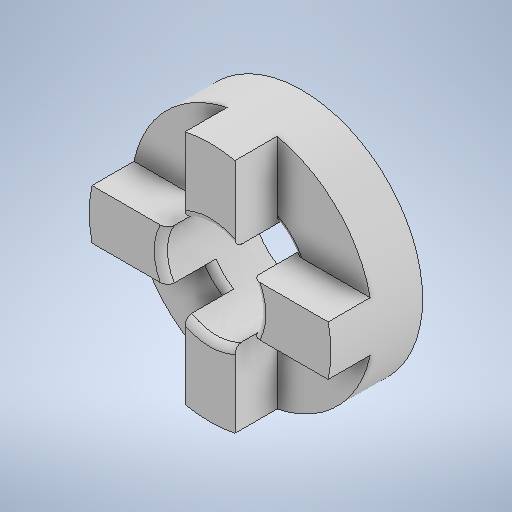
# Autodesk Inventor part: trava_botao_topo
Saved by Autodesk Inventor 2025.3 (Build 293356000, 356)
## iProperties
Created: 2025-07-28
Part Number: trava_botao_topo
Material: Genérico
Document SubType Name: Modeling
Designer: user
Density: 1 g/cm^3
Appearance: Padrão
Author: user
## iProperties of the stored document trava_botao_topo_3DPrint.ipt
Created: 2025-07-28
Part Number: trava_botao_topo_3DPrint
Material: Genérico
Document SubType Name: Modeling
Designer: user
Density: 1 g/cm^3
Appearance: Padrão
Author: user
Autodesk Inventor part; units mm, degrees
ref_plane "YZ Plane" through (0, 0, 0) normal (1, 0, 0) x (0, 1, 0)
ref_plane "XZ Plane" through (0, 0, 0) normal (0, 1, 0) x (-1, 0, 0)
ref_plane "XY Plane" through (0, 0, 0) normal (0, 0, 1) x (1, 0, 0)
sketch "Esboço1" plane through (0, 0, 0) normal (0, 0, 1) x (1, 0, 0)
  circle A0 centre (0, 0) radius 3.75
  circle A1 centre (0, 0) radius 7.2
  circle A2 centre (0, 0) radius 9.2
  dimension "d0" = 7.5
  dimension "d2" = 14.4
  dimension "d3" = 18.4
  constraints: 3 centre point, 3 coincident
  measures "d0" diameter of A0
  measures "d2" diameter of A1
  measures "d3" diameter of A2
extrude "Extrusão1" add sketch "Esboço1" along normal blind 7 contours A1 | A2
sketch "Esboço2" plane through (0, 0, 7) normal (0, 0, 1) x (1, 0, 0)
  circle A0 centre (0, 0) radius 9.2 projected
  line L0 (-9.2, 1.9) -> (-9.2, -1.9)
  line L1 (-1.9, 9.2) -> (1.9, 9.2)
  line L2 (9.2, 1.9) -> (9.2, -1.9)
  line L3 (-1.9, -9.2) -> (1.9, -9.2)
  line L4 (-1.9, 9.2) -> (-1.9, 3.1165)
  line L5 (-1.9, -3.1165) -> (-1.9, -9.2)
  line L6 (1.9, 9.2) -> (1.9, 3.1165)
  line L7 (1.9, -3.1165) -> (1.9, -9.2)
  line L8 (-9.2, -1.9) -> (-3.1165, -1.9)
  line L9 (3.1165, -1.9) -> (9.2, -1.9)
  line L10 (-9.2, 1.9) -> (-3.1165, 1.9)
  line L11 (3.1165, 1.9) -> (9.2, 1.9)
  arc A1 (-3.1165, -1.9) -> (-1.9, -3.1165) centre (0, 0) ccw
  arc A2 (1.9, -3.1165) -> (3.1165, -1.9) centre (0, 0) ccw
  arc A3 (3.1165, 1.9) -> (1.9, 3.1165) centre (0, 0) ccw
  arc A4 (-1.9, 3.1165) -> (-3.1165, 1.9) centre (0, 0) ccw
  point P0 (9.0017, 1.9)
  point P1 (1.9, 9.0017)
  point P2 (1.9, -9.0017)
  point P3 (9.0017, -1.9)
  point P4 (-9.0017, -1.9)
  point P5 (-1.9, -9.0017)
  point P6 (-1.9, 9.0017)
  point P7 (-9.0017, 1.9)
  constraints: 24 end point, 8 point on circle, 4 centre point, 3 perpendicular, 1 coincident, 1 vertical
extrude "Extrusão2" cut sketch "Esboço2" against normal blind 3.2 contours L11 A3 L6 A0 | A0 L7 A2 L9 | L4 A4 L10 A0 | A0 L8 A1 L5
fillet "Arredondamento1" radius 0.5 9 edges at (-3.75, 0, 7) (0, 3.75, 7) (3.6185, -0.9845, 7) (3.6185, 0.9845, 7) (0, -3.75, 7) (-2.6517, -2.6517, 3.8) (-2.6517, 2.6517, 3.8) (2.6517, 2.6517, 3.8) (2.6517, -2.6517, 3.8)
